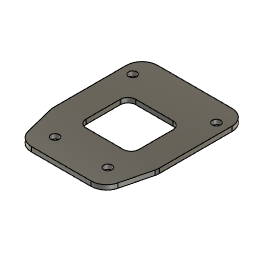
X Axis Support - Inside Support (Autodesk Fusion 360 design; units mm, degrees)
Autodesk Fusion 360 part; units mm, degrees
sketch "Sketch1" plane through (0, 0, 0) normal (0, 0, 1) x (1, 0, 0) in component "X Axis Support - Inside Support"
  line L0 (0, 0) -> (68, 0)
  line L1 (68, 0) -> (68, 86)
  line L2 (68, 86) -> (0, 86)
  line L3 (0, 86) -> (0, 0)
  dimension "d1" = 68
  dimension "d2" = 86
  constraint horizontal L0
  constraint vertical L1
  constraint horizontal L2
  constraint vertical L3
  constraint coincident L0.start L3.end
  measures "d1" distance of L0.start L0.end
  measures "d2" distance of L0.start L2.end
extrude "Extrude1" add sketch "Sketch1" along normal blind 3 in component "X Axis Support - Inside Support"
sketch "Sketch2" plane through (0, 0, 3) normal (0, 0, 1) x (-1, 0, 0) in component "X Axis Support - Inside Support"
  line L0 (0, -86) -> (0, 0)
  line L1 (0, 0) -> (-68, 0)
  line L2 (-68, 0) -> (-68, -86)
  line L3 (-68, -86) -> (0, -86)
  line L4 (-7, -86) -> (-7, 0) construction
  line L5 (-61, -86) -> (-61, 0) construction
  line L6 (0, -13) -> (-68, -13) construction
  line L7 (0, -73) -> (-68, -73) construction
  circle A0 centre (-7, -73) radius 12 construction
  circle A1 centre (-61, -73) radius 12 construction
  circle A2 centre (-7, -73) radius 2.65
  circle A3 centre (-61, -73) radius 2.65
  line L8 (0, -73) -> (0, 0)
  line L9 (0, 0) -> (-34, 0)
  line L10 (-34, 0) -> (-68, 0)
  line L11 (-68, 0) -> (-68, -73)
  line L12 (-17, 0) -> (-17, -86) construction
  line L13 (-51, 0) -> (-51, -86) construction
  circle A4 centre (-17, -13) radius 12 construction
  circle A5 centre (-51, -13) radius 12 construction
  circle A6 centre (-17, -13) radius 2.65
  circle A7 centre (-51, -13) radius 2.65
  line L14 (0, -28) -> (-68, -28) construction
  line L15 (-7, 0) -> (0, -28)
  line L16 (-61, 0) -> (-68, -28)
  line L17 (-17, -28) -> (-51, -28)
  line L18 (-51, -28) -> (-51, -60)
  line L19 (-51, -60) -> (-17, -60)
  line L20 (-17, -60) -> (-17, -28)
  line L21 (0, -86) -> (-68, -86) construction
  line L22 (-34, -86) -> (-34, 0) construction
  dimension "d8" = 13
  dimension "d13" = 24
  dimension "d14" = 24
  dimension "d16" = 5.3
  dimension "d17" = 5.3
  dimension "d40" = 60
  dimension "d53" = 24
  dimension "d54" = 24
  dimension "d55" = 5.3
  dimension "d56" = 5.3
  dimension "d57" = 28
  dimension "d108" = 34
  dimension "d109" = 32
  dimension "d234" = 13
  dimension "d237" = 54
  dimension "d238" = 27
  dimension "d239" = 34
  dimension "d240" = 17
  constraint coincident L3 L4.start
  constraint coincident L1 L4.end
  constraint perpendicular L1 L4
  constraint coincident L3 L5.start
  constraint coincident L1 L5.end
  constraint perpendicular L1 L5
  constraint coincident L1 L9.end
  constraint coincident L0 L6.start
  constraint coincident L2 L6.end
  constraint perpendicular L2 L6
  constraint coincident L0 L7.start
  constraint coincident L2 L7.end
  constraint perpendicular L2 L7
  constraint coincident L7 A0.centre
  constraint coincident L4 A0.centre
  constraint coincident L7 A1.centre
  constraint coincident L5 A1.centre
  constraint concentric A0 A2
  constraint concentric A1 A3
  constraint coincident L0.end L1.start
  constraint coincident L1.end L2.start
  constraint coincident L9 L12.start
  constraint coincident L3 L12.end
  constraint perpendicular L3 L12
  constraint coincident L10 L13.start
  constraint coincident L3 L13.end
  constraint perpendicular L3 L13
  constraint coincident L12 A4.centre
  constraint coincident L6 A4.centre
  constraint coincident L13 A5.centre
  constraint coincident L6 A5.centre
  constraint concentric A4 A6
  constraint concentric A5 A7
  constraint coincident L8 L14.start
  constraint coincident L11 L14.end
  constraint horizontal L17
  constraint vertical L18
  constraint horizontal L19
  constraint vertical L20
  constraint coincident L14 L17.start
  constraint coincident L12 L17.start
  constraint coincident L0 L3.end
  constraint coincident L2 L3.start
  constraint perpendicular L2 L21
  constraint midpoint L21 L22.start
  constraint perpendicular L9 L22
  measures "d8" distance of L1 L6
  measures "d13" diameter of A0
  measures "d14" diameter of A1
  measures "d16" diameter of A2
  measures "d17" diameter of A3
  measures "d40" distance of L6 L7
  measures "d53" diameter of A4
  measures "d54" diameter of A5
  measures "d55" diameter of A6
  measures "d56" diameter of A7
  measures "d57" distance of L10 L14
  measures "d108" distance of L17.start L17.end
  measures "d109" distance of L17.start L19.end
  measures "d234" distance of A0.centre L21
  measures "d237" distance of L4 L5
  measures "d238" distance of L4 L22
  measures "d239" distance of L12 L13
  measures "d240" distance of L12 L22
extrude "Extrude2" cut sketch "Sketch2" against normal up to surface (3 mm away) contours L0 L1 L8 L9 L15 | L1 L2 L10 L11 L16 | A2 | A3 | A6 | A7 | L17 L18 L19 L20 in component "X Axis Support - Inside Support"
fillet "Fillet5" radius 5 4 edges at (17, 60, 1.5) (51, 60, 1.5) (51, 28, 1.5) (17, 28, 1.5) in component "X Axis Support - Inside Support"
fillet "Fillet5" radius 10 4 edges at (0, 28, 1.5) (7, 0, 1.5) (61, 0, 1.5) (68, 28, 1.5) in component "X Axis Support - Inside Support"
fillet "Fillet5" radius 10 2 edges at (0, 86, 1.5) (68, 86, 1.5) in component "X Axis Support - Inside Support"
sketch "Sketch2 (2)" plane through (0, 0, 3) normal (0, 0, 1) x (-1, 0, 0)
  line L0 (0, -76) -> (0, -29.2311)
  arc A0 (0, -29.2311) -> (-0.2986, -26.8057) centre (-10, -29.2311) ccw
  line L1 (-0.2986, -26.8057) -> (-5.1063, -7.5746)
  arc A1 (-5.1063, -7.5746) -> (-14.8078, 0) centre (-14.8078, -10) ccw
  line L2 (-14.8078, 0) -> (-53.1922, 0)
  arc A2 (-53.1922, 0) -> (-62.8937, -7.5746) centre (-53.1922, -10) ccw
  line L3 (-62.8937, -7.5746) -> (-67.7014, -26.8057)
  arc A3 (-67.7014, -26.8057) -> (-68, -29.2311) centre (-58, -29.2311) ccw
  line L4 (-68, -29.2311) -> (-68, -76)
  line L5 (-58, -86) -> (-10, -86)
  line L6 (-22, -60) -> (-46, -60)
  arc A4 (-51, -55) -> (-46, -60) centre (-46, -55) ccw
  line L7 (-51, -55) -> (-51, -33)
  arc A5 (-46, -28) -> (-51, -33) centre (-46, -33) ccw
  line L8 (-46, -28) -> (-22, -28)
  arc A6 (-17, -33) -> (-22, -28) centre (-22, -33) ccw
  line L9 (-17, -33) -> (-17, -55)
  arc A7 (-22, -60) -> (-17, -55) centre (-22, -55) ccw
  circle A8 centre (-17, -13) radius 2.65
  circle A9 centre (-61, -73) radius 2.65
  circle A10 centre (-51, -13) radius 2.65
  circle A11 centre (-7, -73) radius 2.65
  line L10 (-34, -150) -> (-34, -110) construction
  line L11 (-34, -110) -> (-7, -73) construction
  line L12 (-34, -110) -> (-61, -73) construction
  line L13 (-34, -108.4681) -> (-34, -60) construction
  line L14 (-34, -122) -> (-36, -122)
  line L15 (-34, -122) -> (-32, -122)
  line L16 (-34, -142) -> (-36, -142)
  line L17 (-34, -142) -> (-32, -142)
  line L18 (-32, -142) -> (-32, -122)
  line L19 (-36, -142) -> (-36, -122)
  line L20 (-26.9264, -100.3065) -> (-28.542, -99.1276)
  line L21 (-26.9264, -100.3065) -> (-25.3108, -101.4854)
  line L22 (-12.1896, -80.1117) -> (-13.8052, -78.9328)
  line L23 (-12.1896, -80.1117) -> (-10.5741, -81.2907)
  line L24 (-25.3108, -101.4854) -> (-10.5741, -81.2907)
  line L25 (-28.542, -99.1276) -> (-13.8052, -78.9328)
  line L26 (-41.0736, -100.3065) -> (-42.6892, -101.4854)
  line L27 (-41.0736, -100.3065) -> (-39.458, -99.1276)
  line L28 (-55.8104, -80.1117) -> (-57.4259, -81.2907)
  line L29 (-55.8104, -80.1117) -> (-54.1948, -78.9328)
  line L30 (-54.1948, -78.9328) -> (-39.458, -99.1276)
  line L31 (-57.4259, -81.2907) -> (-42.6892, -101.4854)
  line L32 (-34, -98) -> (-36, -98)
  line L33 (-34, -98) -> (-32, -98)
  line L34 (-34, -66) -> (-36, -66)
  line L35 (-34, -66) -> (-32, -66)
  line L36 (-32, -98) -> (-32, -66)
  line L37 (-36, -98) -> (-36, -66)
  arc A12 (-68, -76) -> (-58, -86) centre (-58, -76) ccw
  arc A13 (-10, -86) -> (0, -76) centre (-10, -76) ccw
  dimension "d207" = 2
  dimension "d208" = 2
  dimension "d209" = 12
  dimension "d210" = 2
  dimension "d211" = 2
  dimension "d212" = 20
  dimension "d213" = 2
  dimension "d214" = 2
  dimension "d215" = 12
  dimension "d216" = 2
  dimension "d217" = 2
  dimension "d218" = 25
  dimension "d219" = 2
  dimension "d220" = 2
  dimension "d221" = 2
  dimension "d222" = 2
  dimension "d223" = 12
  dimension "d224" = 25
  dimension "d225" = 2
  dimension "d226" = 2
  dimension "d227" = 12
  dimension "d228" = 2
  dimension "d229" = 2
  dimension "d230" = 32
  constraint coincident A11.centre L11.end
  constraint coincident A9.centre L12.end
  constraint midpoint L6 L13.end
  constraint perpendicular L6 L13
  constraint coincident L10 L14.start
  constraint perpendicular L10 L14
  constraint perpendicular L10 L15
  constraint coincident L10 L16.start
  constraint perpendicular L10 L16
  constraint perpendicular L10 L17
  constraint coincident L11 L20.start
  constraint perpendicular L11 L20
  constraint perpendicular L11 L21
  constraint coincident L11 L22.start
  constraint perpendicular L11 L22
  constraint perpendicular L11 L23
  constraint coincident L12 L26.start
  constraint perpendicular L12 L26
  constraint perpendicular L12 L27
  constraint coincident L12 L28.start
  constraint perpendicular L12 L28
  constraint perpendicular L12 L29
  constraint coincident L13 L32.start
  constraint perpendicular L13 L32
  constraint perpendicular L13 L33
  constraint coincident L13 L34.start
  constraint perpendicular L13 L34
  constraint perpendicular L13 L35
  measures "d207" distance of L14.start L14.end
  measures "d208" distance of L14.start L15.end
  measures "d209" distance of L10.end L14
  measures "d210" distance of L16.start L16.end
  measures "d211" distance of L16.start L17.end
  measures "d212" distance of L14 L16
  measures "d213" distance of L20.start L20.end
  measures "d214" distance of L20.start L21.end
  measures "d215" distance of L10.end L21
  measures "d216" distance of L22.start L22.end
  measures "d217" distance of L22.start L23.end
  measures "d218" distance of L21 L23
  measures "d219" distance of L26.start L26.end
  measures "d220" distance of L26.start L27.end
  measures "d221" distance of L28.start L28.end
  measures "d222" distance of L28.start L29.end
  measures "d223" distance of L10.end L26
  measures "d224" distance of L26 L28
  measures "d225" distance of L32.start L32.end
  measures "d226" distance of L32.start L33.end
  measures "d227" distance of L10.end L32
  measures "d228" distance of L34.start L34.end
  measures "d229" distance of L34.start L35.end
  measures "d230" distance of L32 L34
component "X Axis Support - Inside Support" placed x (1, 0, 0) y (0, 1, 0) z (0, 0, 1) at (0, 0, 0)
named bodies: "X Axis Support - Inside Support"
